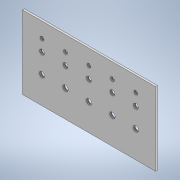
# Autodesk Inventor part: front
Saved by Autodesk Inventor 2021 (Build 250183000, 183)
## iProperties
Created: 2020-07-28
Part Number: front
Material: Generic
Document SubType Name: Modeling
Designer: johna
Density: 1 g/cm^3
Appearance: Default
Author: johna
Autodesk Inventor part; units mm, degrees
ref_plane "YZ Plane" through (0, 0, 0) normal (1, 0, 0) x (0, 1, 0)
ref_plane "XZ Plane" through (0, 0, 0) normal (0, 1, 0) x (-1, 0, 0)
ref_plane "XY Plane" through (0, 0, 0) normal (0, 0, 1) x (1, 0, 0)
sketch "Sketch1" plane through (0, 0, 0) normal (0, 0, 1) x (1, 0, 0)
  line L0 (0, 0) -> (172.72, 0)
  line L1 (172.72, 0) -> (172.72, 95.25)
  line L2 (172.72, 95.25) -> (0, 95.25)
  line L3 (0, 95.25) -> (0, 0)
  dimension "d53" = 172.72
  dimension "d57" = 95.25
  constraints: 8 end point, 2 parallel, 1 horizontal, 1 perpendicular
  measures "d53" distance of L1.end L2.end
  measures "d57" distance of L0.end L1.end
extrude "Extrusion1" add sketch "Sketch1" along normal blind 2.54
sketch "Sketch2" plane through (0, 0, 2.54) normal (0, 0, 1) x (1, 0, 0)
  circle A0 centre (25.4, 35.121) radius 3.5
  circle A1 centre (25.4, 60.521) radius 3.175
  line L0 (0, 95.25) -> (0, 0) projected
  circle A2 centre (55.88, 60.521) radius 3.175
  circle A3 centre (86.36, 60.521) radius 3.175
  circle A4 centre (116.84, 60.521) radius 3.175
  circle A5 centre (147.32, 60.521) radius 3.175
  circle A6 centre (25.4, 75.761) radius 2.5
  circle A7 centre (55.88, 75.761) radius 2.5
  circle A8 centre (86.36, 75.761) radius 2.5
  circle A9 centre (116.84, 75.761) radius 2.5
  circle A10 centre (147.32, 75.761) radius 2.5
  circle A11 centre (55.88, 35.121) radius 3.5
  circle A12 centre (86.36, 35.121) radius 3.5
  circle A13 centre (116.84, 35.121) radius 3.5
  circle A14 centre (147.32, 35.121) radius 3.5
  line L1 (172.72, 0) -> (172.72, 95.25) projected
  dimension "d4" = 7
  dimension "d5" = 6.35
  dimension "d8" = 25.4
  dimension "d9" = 6.35
  dimension "d10" = 6.35
  dimension "d11" = 6.35
  dimension "d12" = 6.35
  dimension "d18" = 0
  dimension "d19" = 0
  dimension "d20" = 0
  dimension "d21" = 0
  dimension "d22" = 5
  dimension "d23" = 15.24
  dimension "d24" = 0
  dimension "d25" = 5
  dimension "d26" = 5
  dimension "d27" = 5
  dimension "d28" = 5
  dimension "d29" = 15.24
  dimension "d34" = 15.24
  dimension "d35" = 15.24
  dimension "d36" = 15.24
  dimension "d37" = 7
  dimension "d38" = 7
  dimension "d39" = 7
  dimension "d40" = 7
  dimension "d41" = 30.48
  dimension "d42" = 25.4
  dimension "d43" = 30.48
  dimension "d44" = 25.4
  dimension "d45" = 30.48
  dimension "d46" = 25.4
  dimension "d47" = 30.48
  dimension "d48" = 25.4
  dimension "d49" = 30.48
  dimension "d50" = 30.48
  dimension "d51" = 30.48
  dimension "d52" = 30.48
  dimension "d58" = 30.48
  dimension "d59" = 30.48
  dimension "d60" = 30.48
  dimension "d61" = 30.48
  dimension "d62" = 0
  dimension "d63" = 25.4
  constraints: 15 centre point
  measures "d4" diameter of A0
  measures "d5" diameter of A1
  measures "d8" distance of A1.centre A0.centre
  measures "d9" diameter of A2
  measures "d10" diameter of A3
  measures "d11" diameter of A4
  measures "d12" diameter of A5
  measures "d18" vertical distance of A3.centre A2.centre
  measures "d19" vertical distance of A1.centre A2.centre
  measures "d20" vertical distance of A3.centre A4.centre
  measures "d21" vertical distance of A4.centre A5.centre
  measures "d22" diameter of A6
  measures "d23" distance of A1.centre A6.centre
  measures "d24" horizontal distance of A1.centre A6.centre
  measures "d25" diameter of A7
  measures "d26" diameter of A8
  measures "d27" diameter of A9
  measures "d28" diameter of A10
  measures "d29" distance of A2.centre A7.centre
  measures "d34" distance of A5.centre A10.centre
  measures "d35" distance of A4.centre A9.centre
  measures "d36" distance of A3.centre A8.centre
  measures "d37" diameter of A11
  measures "d38" diameter of A12
  measures "d39" diameter of A13
  measures "d40" diameter of A14
  measures "d41" distance of A0.centre A11.centre
  measures "d42" distance of A2.centre A11.centre
  measures "d43" distance of A11.centre A12.centre
  measures "d44" distance of A3.centre A12.centre
  measures "d45" distance of A12.centre A13.centre
  measures "d46" distance of A13.centre A4.centre
  measures "d47" distance of A14.centre A13.centre
  measures "d48" distance of A14.centre A5.centre
  measures "d49" distance of A7.centre A6.centre
  measures "d50" distance of A8.centre A7.centre
  measures "d51" distance of A9.centre A8.centre
  measures "d52" distance of A10.centre A9.centre
  measures "d58" distance of A2.centre A1.centre
  measures "d59" distance of A3.centre A2.centre
  measures "d60" distance of A4.centre A3.centre
  measures "d61" distance of A5.centre A4.centre
  measures "d62" horizontal distance of A1.centre A0.centre
  measures "d63" distance from line of L0 A1.centre
extrude "Extrusion2" cut sketch "Sketch2" against normal blind 2.54
body "Solid1"
